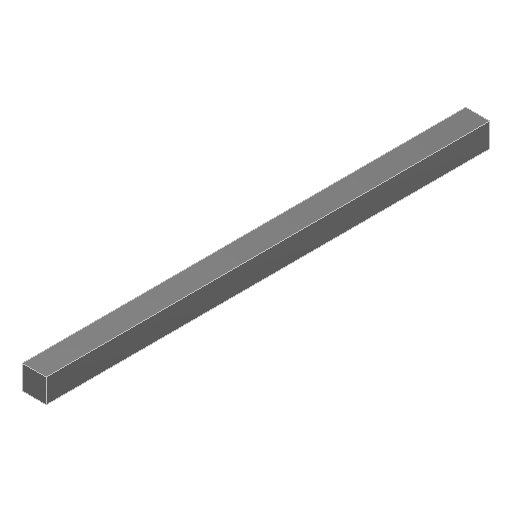
# Autodesk Inventor part: VEJ-00-014
Saved by Autodesk Inventor 2026.1 (Build 301233000, 233)
## iProperties
Company: Venttos
Created: 2025-08-16
Part Number: VEJ-00-014
Material: Durastone BK
Document SubType Name: Modeling
Designer: Willian Pinheiro
Mass: 35.0012 g
Surface Area: 77.2519 cm^2
Volume: 18.4217 cm^3
Density: 1.9 g/cm^3
Appearance: Suave - Preto
Description: Lateral B Palete
Project: VEJ-00
Checked By: Antonio Lucas
Engr Approved By: Antonio Lucas
Mfg Approved By: Anderson Oliveira
Dimensões: 10 x 10 x 185 mm
Total: 2
Author: Willian Pinheiro
Revision Number: 00
Title: Palete
Autodesk Inventor part; units mm, degrees
ref_plane "YZ Plane" through (0, 0, 0) normal (1, 0, 0) x (0, 1, 0)
ref_plane "XZ Plane" through (0, 0, 0) normal (0, 1, 0) x (-1, 0, 0)
ref_plane "XY Plane" through (0, 0, 0) normal (0, 0, 1) x (1, 0, 0)
sketch "Esboço1" plane through (0, 0, 0) normal (0, 0, 1) x (1, 0, 0)
  line L0 (-7, 0) -> (7, 0) construction
  line L1 (0, -129.5) -> (0, 129.5) construction
  line L2 (-5, 92.5) -> (5, 92.5)
  line L3 (5, 92.5) -> (5, -92.5)
  line L4 (5, -92.5) -> (-5, -92.5)
  line L5 (-5, -92.5) -> (-5, 92.5)
  point P0 (0, 0)
  point P1 (0, -67.5)
  point P2 (0, 0)
  point P3 (0, 67.5)
  dimension "d0" = 10
  dimension "d1" = 185
  dimension "d4" = 67.5
  constraints: 8 end point, 2 parallel, 1 coincident, 1 horizontal, 1 perpendicular, 1 point on line, 1 symmetric about line, 2 other
  measures "d0" distance between parallel lines of L3 L5
  measures "d1" distance of L4.end L2.start
  measures "d4" distance of point (0, 0) point (0, -67.5)
extrude "Extrusão1" add sketch "Esboço1" along normal blind 10
hole "Furo1" at (0, -67.5, 0) at (0, 67.5, 0) direction (0, 0, 1) diameter 2.459 depth 8 tip angle 118 thread size "M3x0.5" class "6H" standard "ISO Metric profile"
equation "\"d2\" = d0"
